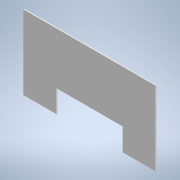
# Autodesk Inventor part: plexiglass3
Saved by Autodesk Inventor 2021 (Build 250183000, 183)
## iProperties
Created: 2021-03-25
Part Number: plexiglass3
Material: Generic
Document SubType Name: Modeling
Designer: con_c_000
Density: 1 g/cm^3
Appearance: Default
Author: con_c_000
Autodesk Inventor part; units mm, degrees
ref_plane "YZ Plane" through (0, 0, 0) normal (1, 0, 0) x (0, 1, 0)
ref_plane "XZ Plane" through (0, 0, 0) normal (0, 1, 0) x (-1, 0, 0)
ref_plane "XY Plane" through (0, 0, 0) normal (0, 0, 1) x (1, 0, 0)
sketch "Sketch1" plane through (0, 0, 0) normal (0, 0, 1) x (1, 0, 0)
  line L0 (-279.4413, 536.8851) -> (-203.2413, 536.8851)
  line L1 (-203.2413, 536.8851) -> (-203.2413, 708.9317)
  line L2 (-203.2413, 708.9317) -> (-279.4413, 708.9317)
  line L3 (-279.4413, 708.9317) -> (-279.4413, 536.8851)
  line L4 (-203.2413, 708.9317) -> (-49.5365, 708.9317)
  line L5 (-49.5365, 708.9317) -> (-49.5365, 588.8786)
  line L6 (-49.5365, 588.8786) -> (-203.2413, 588.8786)
  line L7 (-203.2413, 588.8786) -> (-203.2413, 708.9317)
  line L8 (-49.5365, 708.9317) -> (26.6635, 708.9317)
  line L9 (26.6635, 708.9317) -> (26.6635, 536.8851)
  line L10 (26.6635, 536.8851) -> (-49.5365, 536.8851)
  line L11 (-49.5365, 536.8851) -> (-49.5365, 708.9317)
  point P0 (0, 0)
  dimension "d0" = 76.2
  dimension "d1" = 76.2
  constraints: 24 end point, 6 parallel, 3 horizontal, 3 perpendicular
  measures "d0" distance of L2.end L1.end
  measures "d1" distance of L9.end L10.end
extrude "Extrusion1" add sketch "Sketch1" along normal blind 2.54
body "Solid1"
